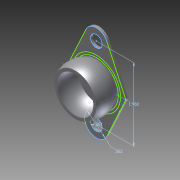
# Autodesk Inventor part: Misc_FlangeMount_Triangle_4050
Saved by Autodesk Inventor 2013 (Build 170138000, 138)
## iProperties
Category: Miscellaneous
Company: Autodesk Inc.
Created: 2012-12-03
Part Number: Misc_FlangeMount_Triangle_4050
Document SubType Name: Modeling
Designer: Autodesk Inc.
Density: 1 g/cm^3
Material: Generic
Author: Autodesk Inc.
Autodesk Inventor part; units mm, degrees
ref_plane "YZ Plane" through (0, 0, 0) normal (1, 0, 0) x (0, 1, 0)
ref_plane "XZ Plane" through (0, 0, 0) normal (0, 1, 0) x (-1, 0, 0)
ref_plane "XY Plane" through (0, 0, 0) normal (0, 0, 1) x (1, 0, 0)
sketch "Sketch1" plane through (0, 0, 0) normal (0, 0, 1) x (1, 0, 0)
  circle A0 centre (0, 0) radius 3.5687
  arc A1 (-6.4809, -2.9901) -> (6.4801, -2.9918) centre (0, 0) ccw
  line L0 (-20.3315, 22.225) -> (23.7148, 22.225)
  circle A2 centre (0, 44.45) radius 3.5687
  arc A3 (6.4801, 47.4418) -> (-6.4809, 47.4401) centre (0, 44.45) ccw
  circle A4 centre (0, 22.225) radius 14.8487
  circle A5 centre (0, 22.225) radius 13.5003
  line L1 (-18.1146, 22.225) -> (-6.4809, 47.4401)
  line L2 (18.1226, 22.225) -> (6.4801, 47.4418)
  line L3 (-18.1146, 22.225) -> (-6.4809, -2.9901)
  line L4 (18.1226, 22.225) -> (6.4801, -2.9918)
  point P0 (-14.3353, 14.0338)
  point P1 (14.3408, 14.0338)
  dimension "d0" = 7.1374
  dimension "d1" = 14.2748
  dimension "d2" = 44.45
  constraints: 10 end point, 6 centre point, 5 coincident, 5 point on line, 4 point on circle, 4 tangent, 3 symmetric about line, 2 equal length, 1 horizontal, 1 horizontal alignment, 2 other
  measures "d0" diameter of A0
  measures "d1" diameter of A1
  measures "d2" distance of A2.centre A0.centre
extrude "Extrusion1" add sketch "Sketch1" against normal blind 1.6002
sketch "Sketch2" plane through (0, 0, 0) normal (1, 0, 0) x (0, 1, 0)
  point P0 (0, 0)
sketch "Sketch3" plane through (0, 0, 0) normal (1, 0, 0) x (0, 1, 0)
  arc A0 (35.7382, 2.1018) -> (35.0472, 13.022) centre (22.225, 6.7287) ccw
  line L0 (51.5874, 0) -> (47.4401, 0) projected
  line L1 (51.5874, 0) -> (34.4832, 0)
  line L2 (-2.9901, 0) -> (-7.1374, 0) projected
  line L3 (-7.1374, 0) -> (7.1476, 1.1293)
  line L4 (33.3323, 12.8864) -> (35.0472, 13.022)
  arc A1 (35.7382, 2.1018) -> (37.2401, 0) centre (37.2401, 1.5875) ccw
  line L5 (48.0187, -1.6002) -> (40.8813, -1.6002) projected
  line L6 (3.5687, -1.6002) -> (-3.5687, -1.6002) projected
  line L7 (22.225, -1.6002) -> (-2.9901, -1.6002) projected
  line L8 (47.4401, -1.6002) -> (22.225, -1.6002) projected
  line L9 (47.4418, -1.6002) -> (47.4401, -1.6002) projected
  line L10 (22.225, -1.6002) -> (47.4418, -1.6002) projected
  line L11 (-2.9918, -1.6002) -> (22.225, -1.6002) projected
  line L12 (-2.9901, -1.6002) -> (-2.9918, -1.6002) projected
  arc A2 (34.2371, 2.6056) -> (33.3323, 12.8864) centre (22.225, 6.7287) ccw
  line L13 (51.5874, -1.6002) -> (47.4401, -1.6002) projected
  line L14 (51.5874, -1.6002) -> (37.2401, -1.6002)
  arc A3 (34.2371, 2.6056) -> (34.4832, 0) centre (37.2401, 1.5748) ccw
  line L15 (22.225, -1.6002) -> (22.225, 16.2984)
  arc A4 (34.4832, 0) -> (37.2401, -1.6002) centre (37.2401, 1.5748) ccw
  line L16 (37.2401, -1.6002) -> (22.225, -1.6002)
  line L17 (34.4832, 0) -> (22.225, 0)
  point P0 (0, 0)
  point P1 (47.4418, 0)
  point P2 (-2.9918, 0)
  point P3 (31.8125, -1.6002)
  dimension "d28" = 1.5875
  dimension "d29" = 3.175
  constraints: 14 end point, 11 point on circle, 7 tangent, 5 centre point, 5 point on line, 3 perpendicular, 2 collinear, 2 other
  measures "d28" radius of A1
  measures "d29" radius of A3
revolve "Revolution2" add sketch "Sketch3" angle 360 about axis through (0, 22.225, -1.6002) along (0, 0, 1) contours A1 L1 A3 A2 L4 A0
revolve "Revolution3" cut sketch "Sketch3" angle 360 about axis through (0, 22.225, -1.6002) along (0, 0, 1) contours A4 L8 L15 L17
sketch "Sketch4" plane through (0, 0, 0) normal (0, 0, 1) x (1, 0, 0)
  line L0 (6.4801, -2.9918) -> (18.1226, 22.225) projected
  line L1 (18.1226, 22.225) -> (6.4801, 47.4418) projected
  circle A0 centre (0, 44.45) radius 3.5687 projected
  circle A1 centre (0, 22.225) radius 15.0151 projected
  line L2 (0, 44.45) -> (0, 57.4596)
  line L3 (-14.2875, 44.45) -> (-14.2875, 57.4596)
  arc A2 (14.2875, 30.5316) -> (14.2875, 26.8424) centre (18.632, 28.687) ccw
  arc A3 (14.2875, 17.6076) -> (14.2875, 26.8424) centre (0, 22.225) ccw
  arc A4 (14.2875, 17.6076) -> (14.2875, 13.9184) centre (18.632, 15.763) ccw
  line L4 (14.2875, 30.5316) -> (14.2875, 57.4596)
  dimension "d33" = 14.2875
  constraints: 8 point on circle, 6 end point, 3 centre point, 2 equal radius, 2 parallel, 2 point on line, 1 vertical
  measures "d33" distance between parallel lines of L3 L2
extrude "Extrusion2" cut sketch "Sketch4" against normal up to next contours A4 A1 A2 L1 L0 | A4 A1 | A1 A2
mirror "Mirror1" about plane through (0, 0, 0) normal (1, 0, 0) of "Extrusion2"
equation "\"d33\" = 0.5 * d32"
equation "\"d32\" = 28.575"
body "Solid1"
